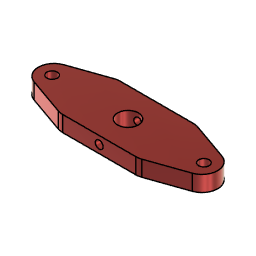
Handlebar v10 (Autodesk Fusion 360 design; units mm, degrees)
Autodesk Fusion 360 part; units mm, degrees
sketch "Main" plane through (0, 0, 0) normal (0, 0, 1) x (1, 0, 0)
  line L0 (-7.5, 5.5) -> (7.5, 5.5)
  line L1 (7.5, 5.5) -> (17.5, 2)
  line L2 (17.5, 2) -> (17.5, -2)
  line L3 (17.5, -2) -> (7.5, -5.5)
  line L4 (7.5, -5.5) -> (-7.5, -5.5)
  line L5 (-7.5, -5.5) -> (-17.5, -2)
  line L6 (-17.5, -2) -> (-17.5, 2)
  line L7 (-17.5, 2) -> (-7.5, 5.5)
  circle A0 centre (0, 0) radius 2
  dimension "d1" = 4
  dimension "d2" = 15
  dimension "d3" = 15
  dimension "d4" = 7.5
  dimension "d5" = 5.5
  dimension "d6" = 5.5
  dimension "d7" = 10
  dimension "d8" = 10
  dimension "d9" = 4
  dimension "d10" = 4
  dimension "d11" = 3.5
  constraint horizontal L0
  constraint perpendicular L0 L2
  constraint parallel L0 L4
  constraint parallel L1 L5
  constraint perpendicular L4 L6
  constraint coincident A0.centre origin
  constraint vertical L0.start L4.end
  measures "d1" diameter of A0
  measures "d2" distance of L0.start L0.end
  measures "d3" distance of L3.end L4.end
  measures "d4" horizontal distance of A0.centre L0.start
  measures "d5" distance of L0 A0.centre
  measures "d6" distance of L4 A0.centre
  measures "d7" distance of L4.end L6
  measures "d8" distance of L2 L3.end
  measures "d9" distance of L5.end L6.end
  measures "d10" distance of L1.end L2.end
  measures "d11" vertical distance of L0.start L6.end
extrude "Extrude1" add sketch "Main" along normal blind 3
sketch "Face holes" plane through (0, 0, 3) normal (0, 0, 1) x (-1, 0, 0)
  circle A0 centre (0, 0) radius 2
  line L0 (17.5, -2) -> (17.5, 2)
  line L1 (17.5, 2) -> (7.5, 5.5)
  line L2 (7.5, 5.5) -> (-7.5, 5.5)
  line L3 (-7.5, 5.5) -> (-17.5, 2)
  line L4 (-17.5, 2) -> (-17.5, -2)
  line L5 (-17.5, -2) -> (-7.5, -5.5)
  line L6 (-7.5, -5.5) -> (7.5, -5.5)
  line L7 (7.5, -5.5) -> (17.5, -2)
  circle A1 centre (14.5, 0) radius 1
  circle A2 centre (-14.5, 0) radius 1
  dimension "d14" = 2
  dimension "d15" = 2
  dimension "d16" = 29
  dimension "d18" = 14.5
  constraint horizontal A0.centre A2.centre
  constraint horizontal A0.centre A1.centre
  measures "d14" diameter of A1
  measures "d15" diameter of A2
  measures "d16" horizontal distance of A1.centre A2.centre
  measures "d18" distance of A0.centre A1.centre
extrude "Extrude2" cut sketch "Face holes" against normal blind 3 contours A1 | A2
fillet "Fillet1" radius 3 8 edges at (-17.5, -2, 1.5) (-7.5, -5.5, 1.5) (7.5, -5.5, 1.5) (17.5, -2, 1.5) (17.5, 2, 1.5) (7.5, 5.5, 1.5) (-7.5, 5.5, 1.5) (-17.5, 2, 1.5)
sketch "Hole Pin" plane through (0, -5.5, 0) normal (0, -1, 0) x (1, 0, 0)
  line L0 (6.9902, 0) -> (6.9902, 3)
  line L1 (6.9902, 3) -> (-6.9902, 3)
  line L2 (-6.9902, 3) -> (-6.9902, 0)
  line L3 (-6.9902, 0) -> (6.9902, 0)
  circle A0 centre (0, 1.5) radius 0.75
  dimension "d23" = 1.5
  dimension "d24" = 1.5
  constraint vertical origin A0.centre
  measures "d23" diameter of A0
  measures "d24" distance of L1 A0.centre
extrude "Extrude3" cut sketch "Hole Pin" against normal blind 17 contours A0
